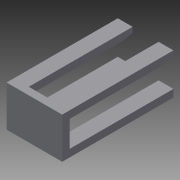
# Autodesk Inventor part: SoporteFio
Saved by Autodesk Inventor 2013 (Build 170138000, 138)
## iProperties
Created: 2013-05-06
Part Number: SoporteFio
Material: Generic
Document SubType Name: Modeling
Designer: otrab
Density: 1 g/cm^3
Author: otrab
Autodesk Inventor part; units mm, degrees
ref_plane "YZ Plane" through (0, 0, 0) normal (1, 0, 0) x (0, 1, 0)
ref_plane "XZ Plane" through (0, 0, 0) normal (0, 1, 0) x (-1, 0, 0)
ref_plane "XY Plane" through (0, 0, 0) normal (0, 0, 1) x (1, 0, 0)
sketch "Sketch1" plane through (0, 0, 0) normal (0, 1, 0) x (-1, 0, 0)
  line L0 (-7.5, -5.5) -> (7.5, -5.5)
  line L1 (7.5, -5.5) -> (7.5, 5.5)
  line L2 (7.5, 5.5) -> (-7.5, 5.5)
  line L3 (-7.5, 5.5) -> (-7.5, -5.5)
  line L4 (-7.5, -5.5) -> (7.5, 5.5) construction
  line L5 (7.5, -5.5) -> (-7.5, 5.5) construction
  point P0 (0, 0)
  dimension "d0" = 15
  dimension "d1" = 11
  constraints: 12 end point, 2 midpoint, 2 parallel, 1 horizontal, 1 perpendicular
  measures "d0" distance of L2.end L1.end
  measures "d1" distance of L0.end L1.end
extrude "Extrusion1" add sketch "Sketch1" along normal blind 30
sketch "Sketch2" plane through (0, 30, 0) normal (0, 1, 0) x (1, 0, 0)
  line L0 (7.5, 5.5) -> (-7.5, 5.5) projected
  line L1 (7.5, -3.5) -> (-7.5, -3.5)
  line L2 (-7.5, -3.5) -> (-7.5, 3.5)
  line L3 (-7.5, 3.5) -> (7.5, 3.5)
  line L4 (7.5, 3.5) -> (7.5, -3.5)
  line L5 (7.5, -3.5) -> (-7.5, 3.5) construction
  line L6 (-7.5, -3.5) -> (7.5, 3.5) construction
  line L7 (-7.5, 5.5) -> (-7.5, -5.5) projected
  line L8 (3.5, -5.5) -> (-3.5, -5.5)
  line L9 (-3.5, -5.5) -> (-3.5, 5.5)
  line L10 (-3.5, 5.5) -> (3.5, 5.5)
  line L11 (3.5, 5.5) -> (3.5, -5.5)
  line L12 (3.5, -5.5) -> (-3.5, 5.5) construction
  line L13 (-3.5, -5.5) -> (3.5, 5.5) construction
  point P0 (0, 0)
  dimension "d4" = 15
  dimension "d5" = 2
  dimension "d8" = 4
  constraints: 24 end point, 4 midpoint, 4 parallel, 2 horizontal, 2 perpendicular, 1 point on line
  measures "d4" distance of L2.end L3.end
  measures "d5" distance between parallel lines of L0 L3
  measures "d8" distance between parallel lines of L7 L9
extrude "Extrusion2" cut sketch "Sketch2" against normal blind 28 contours L11 L3 L9 L0 | L11 L1 L9 L3 | L3 L4 L1 L11 | L9 L1 L2 L3 | L11 L8 L9 L1
sketch "Sketch3" plane through (7.5, 0, 5.5) normal (1, 0, 0) x (0, 0, -1)
  line L0 (2, 2) -> (2, 30) projected
  line L1 (0, 30) -> (2, 30) projected
  line L2 (1, 30) -> (2, 30) construction
  line L3 (1.5, 30) -> (2, 27.042)
  line L4 (2, 27.042) -> (2, 30)
  line L5 (1.5, 30) -> (2, 30)
  point P0 (5.5, 0)
  dimension "d9" = 3
  constraints: 8 end point, 2 collinear, 2 midpoint, 1 perpendicular, 1 point on line
  measures "d9" distance of L3.start L3.end
extrude "Extrusion3" cut sketch "Sketch3" against normal through all
body "Solid1"
